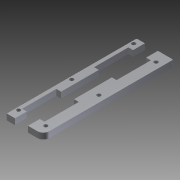
# Autodesk Inventor part: suplemento cojinete
Saved by Autodesk Inventor 2012 SP1 (Build 160190100, 190)
## iProperties
Created: 2014-12-30
Part Number: suplemento cojinete
Material: Default
Document SubType Name: Modeling
Designer: PRINCIPAL
Density: 1 g/cm^3
Author: PRINCIPAL
Autodesk Inventor part; units mm, degrees
ref_plane "YZ Plane" through (0, 0, 0) normal (1, 0, 0) x (0, 1, 0)
ref_plane "XZ Plane" through (0, 0, 0) normal (0, 1, 0) x (-1, 0, 0)
ref_plane "XY Plane" through (0, 0, 0) normal (0, 0, 1) x (1, 0, 0)
sketch "Boceto1" plane through (0, 0, 0) normal (0, 0, 1) x (1, 0, 0)
  line L0 (220, 79) -> (220, 30)
  circle A0 centre (222.5, -17.5085) radius 1.6
  circle A1 centre (222.4918, 27.5) radius 1.6
  circle A2 centre (245.5, 27.5) radius 1.6
  circle A3 centre (245.5, -17.5) radius 1.6
  circle A4 centre (222.4918, 80) radius 1.6
  circle A5 centre (245.5, 75.9891) radius 1.6
  line L1 (220, 30) -> (220, -25)
  line L2 (238, 75) -> (238, 80)
  line L3 (227, 80) -> (227, 75)
  line L4 (220, -25) -> (227, -25)
  line L5 (238, -25) -> (240, -25)
  line L6 (239.9, -15) -> (238, -15)
  line L7 (227, -15) -> (225.1, -15)
  line L8 (227, 41) -> (227, 14)
  line L9 (227, -15) -> (227, -25)
  line L10 (238, -25) -> (238, -15)
  line L11 (238, 14) -> (238, 41)
  line L12 (225.1, 14) -> (227, 14)
  line L13 (238, 14) -> (239.9, 14)
  line L14 (225.1, -15) -> (223, -15)
  line L15 (239.9, -15) -> (242, -15)
  line L16 (225.1, 14) -> (223, 14)
  line L17 (239.9, 14) -> (242, 14)
  line L18 (223, 46) -> (223, 70)
  line L19 (242, 70) -> (242, 46)
  line L20 (223, -15) -> (223, 14)
  line L21 (242, 14) -> (242, -15)
  line L22 (251, 80) -> (251, -25)
  line L23 (240, -25) -> (251, -25)
  line L24 (220, 79) -> (220, 85)
  line L25 (227, 80) -> (227, 85)
  line L26 (238, 80) -> (238, 85)
  line L27 (251, 80) -> (251, 85)
  line L28 (251, 85) -> (238, 85)
  line L29 (227, 85) -> (220, 85)
  line L30 (227, 41) -> (227, 46)
  line L31 (238, 41) -> (238, 46)
  line L32 (242, 46) -> (238, 46)
  line L33 (227, 46) -> (223, 46)
  line L34 (223, 70) -> (223, 75)
  line L35 (242, 70) -> (242, 75)
  line L36 (242, 75) -> (238, 75)
  line L37 (227, 75) -> (223, 75)
  dimension "d6" = 7
  dimension "d17" = 7.5
  dimension "d18" = 5
  dimension "d21" = 7.5
  dimension "d22" = 7.5
  dimension "d23" = 4.5082
  dimension "d24" = 4.5
  constraints: 76 end point, 21 parallel, 19 perpendicular, 6 centre point, 2 collinear
  measures "d6" distance between parallel lines of L1 L8
  measures "d17" distance from line of L2 A5.centre
  measures "d18" distance from line of A4.centre L29
  measures "d21" distance from line of L11 A2.centre
  measures "d22" distance from line of L10 A3.centre
  measures "d23" distance from line of A1.centre L8
  measures "d24" distance from line of A0.centre L9
extrude "Extrusión1" add sketch "Boceto1" along normal blind 5
fillet "Empalme2" radius 5 1 edges at (251, -25, 2.5)
fillet "Empalme3" radius 1 1 edges at (251, 85, 2.5)
fillet "Empalme4" radius 1 1 edges at (220, 85, 2.5)
